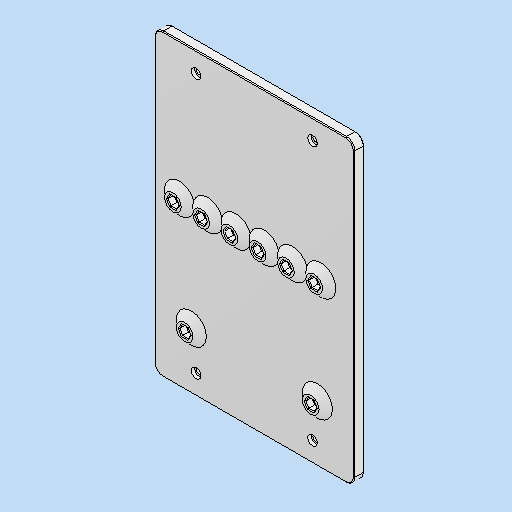
# Autodesk Inventor part: tc-bottom-tray
Saved by Autodesk Inventor 2026 (Build 300175050, 175E)
## iProperties
Created: 2025-06-05
Part Number: tc-bottom-tray
Material: ABS Plastic
Document SubType Name: Modeling
Designer: queezz
Density: 1.06 g/cm^3
Appearance: Smooth - White
Author: queezz
Autodesk Inventor part; units mm, degrees
ref_plane "YZ Plane" through (0, 0, 0) normal (1, 0, 0) x (0, 1, 0)
ref_plane "XZ Plane" through (0, 0, 0) normal (0, 1, 0) x (-1, 0, 0)
ref_plane "XY Plane" through (0, 0, 0) normal (0, 0, 1) x (1, 0, 0)
sketch "Sketch1" plane through (0, 0, 0) normal (0, 0, 1) x (1, 0, 0)
  line L0 (-60, 90) -> (60, 90)
  line L1 (60, 90) -> (60, -90)
  line L2 (60, -90) -> (-60, -90)
  line L3 (-60, -90) -> (-60, 90)
  point P0 (0, 0)
  point P1 (60, 0)
  point P2 (0, 90)
  dimension "d0" = 120
  dimension "d1" = 180
  constraints: 8 end point, 2 midpoint, 2 parallel, 1 horizontal, 1 horizontal alignment, 1 perpendicular, 1 vertical alignment
  measures "d0" distance of L0.start L0.end
  measures "d1" distance of L0.end L1.end
extrude "Extrusion1" add sketch "Sketch1" along normal blind 6
fillet "Fillet1" radius 5 4 edges at (-60, 90, 3) (60, 90, 3) (60, -90, 3) (-60, -90, 3)
chamfer "Chamfer2" distance 0.5 angle 45 16 edges at (0, 90, 6) (-58.5355, 88.5355, 6) (-60, 0, 6) (-58.5355, -88.5355, 6) (0, -90, 6) (58.5355, -88.5355, 6) (60, 0, 6) (58.5355, 88.5355, 6) (0, 90, 0) (-58.5355, 88.5355, 0) (-60, 0, 0) (-58.5355, -88.5355, 0) (0, -90, 0) (58.5355, -88.5355, 0) (60, 0, 0) (58.5355, 88.5355, 0)
sketch "Sketch4" plane through (0, 0, 6) normal (0, 0, 1) x (1, 0, 0)
  line L0 (-35, -78) -> (35, -78) construction
  line L1 (-55, -90) -> (55, -90) projected
  line L2 (-35, 78) -> (35, 78) construction
  line L3 (55, 90) -> (-55, 90) projected
  point P0 (0, 0)
  point P1 (0, -78)
  point P2 (0, 78)
  dimension "d20" = 12
  dimension "d21" = 70
  dimension "d30" = 12
  constraints: 4 coincident, 4 end point, 2 horizontal, 2 midpoint, 2 vertical alignment, 1 parallel
  measures "d20" distance between parallel lines of L1 L0
  measures "d21" distance of L0.start L0.end
  measures "d30" distance between parallel lines of L3 L2
hole "Hole1" at (-35, -78, 6) at (35, -78, 6) at (-35, 78, 6) at (35, 78, 6) direction (0, 0, -1) diameter 3.6 end through all counterbore diameter 5.8 counterbore depth 2
sketch "Sketch5" plane through (0, 0, 0) normal (0, 0, -1) x (-1, 0, 0)
  line L0 (55, 90) -> (-55, 90) projected
  point P0 (45, 8)
  point P1 (0, 0)
  dimension "d45" = 82
  dimension "d46" = 45
  measures "d45" distance from line of L0 point (45, 8)
  measures "d46" horizontal distance of point (0, 0) point (45, 8)
hole "Hole2" at (-45, 8, 0) direction (0, 0, 1) diameter 3.6 end through all
sketch "Sketch7" plane through (0, 0, 6) normal (0, 0, 1) x (1, 0, 0)
  circle A0 centre (-45, 8) radius 1.8 projected
  circle A1 centre (-45, 8) radius 5
  line L0 (-46.6743, 5.1) -> (-48.3486, 8)
  line L1 (-48.3486, 8) -> (-46.6743, 10.9)
  line L2 (-46.6743, 10.9) -> (-43.3257, 10.9)
  line L3 (-43.3257, 10.9) -> (-41.6514, 8)
  line L4 (-41.6514, 8) -> (-43.3257, 5.1)
  line L5 (-43.3257, 5.1) -> (-46.6743, 5.1)
  point P0 (0, 0)
  dimension "d47" = 5.8
  dimension "d48" = 10
  constraints: 12 end point, 2 coincident, 1 centre point, 1 horizontal, 13 other
  measures "d47" distance between parallel lines of L2 L5
  measures "d48" diameter of A1
extrude "Extrusion4" add sketch "Sketch7" along normal blind 4 contours A1
chamfer "Chamfer3" distance 4 angle 45 1 edges at (-50, 8, 6)
pattern_linear "Rectangular Pattern1" count 6 spacing 17 along (1, 0, 0) of "Hole2", "Extrusion4", "Chamfer3"
sketch "Sketch6" plane through (0, 0, 0) normal (0, 0, -1) x (-1, 0, 0)
  line L0 (-37.9, -56) -> (37.9, -56) construction
  line L1 (-55, -90) -> (55, -90) projected
  point P0 (0, 0)
  point P1 (0, -56)
  dimension "d43" = 75.8
  dimension "d44" = 34
  constraints: 2 coincident, 2 end point, 1 horizontal, 1 midpoint, 1 vertical alignment
  measures "d43" distance of L0.start L0.end
  measures "d44" distance between parallel lines of L1 L0
hole "Hole3" at (-37.9, -56, 0) at (37.9, -56, 0) direction (0, 0, 1) diameter 3.6 end through all
sketch "Sketch8" plane through (0, 0, 6) normal (0, 0, 1) x (1, 0, 0)
  circle A0 centre (-37.9, -56) radius 1.8 projected
  circle A1 centre (-37.9, -56) radius 5
  line L0 (-36.2257, -53.1) -> (-34.5514, -56)
  line L1 (-34.5514, -56) -> (-36.2257, -58.9)
  line L2 (-36.2257, -58.9) -> (-39.5743, -58.9)
  line L3 (-39.5743, -58.9) -> (-41.2486, -56)
  line L4 (-41.2486, -56) -> (-39.5743, -53.1)
  line L5 (-39.5743, -53.1) -> (-36.2257, -53.1)
  point P0 (0, 0)
  dimension "d64" = 5.8
  dimension "d65" = 10
  constraints: 12 end point, 2 coincident, 1 centre point, 1 horizontal, 13 other
  measures "d64" distance between parallel lines of L2 L5
  measures "d65" diameter of A1
extrude "Extrusion5" add sketch "Sketch8" along normal blind 4 contours A1
chamfer "Chamfer4" distance 4 angle 45 1 edges at (-42.9, -56, 6)
mirror "Mirror2" about plane through (0, 0, 0) normal (1, 0, 0) of "Extrusion5", "Chamfer4"
chamfer "Chamfer5" distance 0.5 angle 45 56 edges at (-37.9, -53.1, 10) (-40.4115, -54.55, 10) (-40.4115, -57.45, 10) (-37.9, -58.9, 10) (-35.3885, -57.45, 10) (-35.3885, -54.55, 10) (-37.9, -57.8, 6) (37.9, -53.1, 10) (35.3885, -54.55, 10) (35.3885, -57.45, 10) (37.9, -58.9, 10) (40.4115, -57.45, 10) (40.4115, -54.55, 10) (37.9, -57.8, 6) (40, 10.9, 10) (37.4885, 9.45, 10) (37.4885, 6.55, 10) (40, 5.1, 10) (42.5115, 6.55, 10) (42.5115, 9.45, 10) (40, 6.2, 6) (23, 10.9, 10) (20.4885, 9.45, 10) (20.4885, 6.55, 10) (23, 5.1, 10) (25.5115, 6.55, 10) (25.5115, 9.45, 10) (23, 6.2, 6) (6, 10.9, 10) (8.5115, 9.45, 10) (8.5115, 6.55, 10) (6, 5.1, 10) (3.4885, 6.55, 10) (3.4885, 9.45, 10) (6, 6.2, 6) (-11, 10.9, 10) (-13.5115, 9.45, 10) (-13.5115, 6.55, 10) (-11, 5.1, 10) (-8.4885, 6.55, 10) (-8.4885, 9.45, 10) (-11, 6.2, 6) (-28, 10.9, 10) (-30.5115, 9.45, 10) (-30.5115, 6.55, 10) (-28, 5.1, 10) (-25.4885, 6.55, 10) (-25.4885, 9.45, 10) (-28, 6.2, 6) (-45, 10.9, 10) (-47.5115, 9.45, 10) (-47.5115, 6.55, 10) (-45, 5.1, 10) (-42.4885, 6.55, 10) (-42.4885, 9.45, 10) (-45, 6.2, 6)
equation "\"d0\" = width"
equation "\"d1\" = hight"
equation "\"hight\" = 180"
equation "\"width\" = 120"
body "Solid1"
